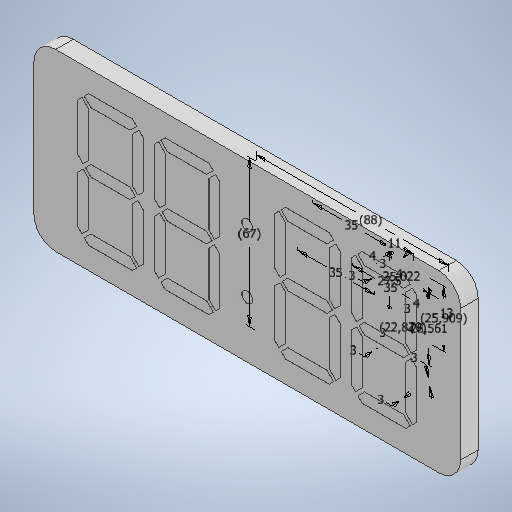
# Autodesk Inventor part: led 7 seg v3
Saved by Autodesk Inventor 2026 (Build 300175000, 175)
## iProperties
Created: 2025-05-20
Part Number: led 7 seg v3
Material: Generic
Document SubType Name: Modeling
Designer: Korobeynikov
Density: 1 g/cm^3
Appearance: Default
Author: Korobeynikov
Autodesk Inventor part; units mm, degrees
ref_plane "YZ Plane" through (0, 0, 0) normal (1, 0, 0) x (0, 1, 0)
ref_plane "XZ Plane" through (0, 0, 0) normal (0, 1, 0) x (-1, 0, 0)
ref_plane "XY Plane" through (0, 0, 0) normal (0, 0, 1) x (1, 0, 0)
sketch "Sketch1" plane through (0, 0, 0) normal (0, 0, 1) x (1, 0, 0)
  line L0 (-94.4527, 39.0647) -> (-94.5898, 54.9894)
  line L1 (-94.5898, 54.9894) -> (-92.9178, 56.6614)
  line L2 (-92.9178, 56.6614) -> (-89.7384, 53.6189)
  line L3 (-89.7384, 53.6189) -> (-89.5199, 39.1071)
  line L4 (-89.5199, 39.1071) -> (-91.8763, 36.6527)
  line L5 (-91.8763, 36.6527) -> (-94.4527, 39.0647)
  line L6 (-91.7267, 57.8164) -> (-89.9627, 59.534)
  line L7 (-89.9627, 59.534) -> (-75.9897, 59.6269)
  line L8 (-75.9897, 59.6269) -> (-74.3185, 57.8164)
  line L9 (-74.3185, 57.8164) -> (-77.2431, 54.8454)
  line L10 (-77.2431, 54.8454) -> (-88.6597, 54.6665)
  line L11 (-88.6597, 54.6665) -> (-91.7267, 57.8164)
  line L12 (-76.2169, 53.8075) -> (-73.4316, 57.0375)
  line L13 (-73.4316, 57.0375) -> (-71.7604, 55.4127)
  line L14 (-71.7604, 55.4127) -> (-71.1618, 39.5726)
  line L15 (-71.1618, 39.5726) -> (-73.39, 36.9729)
  line L16 (-73.39, 36.9729) -> (-75.9897, 39.3869)
  line L17 (-75.9897, 39.3869) -> (-76.2169, 53.8075)
  line L18 (-94.4164, 31.9932) -> (-91.951, 34.3514)
  line L19 (-91.951, 34.3514) -> (-89.4141, 31.9932)
  line L20 (-89.4141, 31.9932) -> (-89.2355, 17.2723)
  line L21 (-89.2355, 17.2723) -> (-92.344, 14.0208)
  line L22 (-92.344, 14.0208) -> (-94.4164, 15.5572)
  line L23 (-94.4164, 15.5572) -> (-94.4164, 31.9932)
  line L24 (-75.7293, 32.3505) -> (-73.4426, 34.7802)
  line L25 (-73.4426, 34.7802) -> (-71.1201, 32.3505)
  line L26 (-71.1201, 32.3505) -> (-70.5842, 16.4505)
  line L27 (-70.5842, 16.4505) -> (-72.2278, 14.4496)
  line L28 (-72.2278, 14.4496) -> (-75.4792, 17.5581)
  line L29 (-75.4792, 17.5581) -> (-75.7293, 32.3505)
  line L30 (-91.32, 13.0418) -> (-88.1993, 16.0932)
  line L31 (-88.1993, 16.0932) -> (-76.5869, 16.4862)
  line L32 (-76.5869, 16.4862) -> (-73.4783, 13.3777)
  line L33 (-73.4783, 13.3777) -> (-75.0147, 11.6269)
  line L34 (-75.0147, 11.6269) -> (-89.3605, 11.0378)
  line L35 (-89.3605, 11.0378) -> (-91.32, 13.0418)
  line L36 (-120.187, 34.9851) -> (-117.7903, 37.3494)
  line L37 (-117.7903, 37.3494) -> (-105.9036, 37.6409)
  line L38 (-105.9036, 37.6409) -> (-103.4421, 35.309)
  line L39 (-103.4421, 35.309) -> (-106.0008, 32.8474)
  line L40 (-106.0008, 32.8474) -> (-117.8069, 32.5723)
  line L41 (-117.8069, 32.5723) -> (-120.187, 34.9851)
  line L42 (-90.8505, 35.6062) -> (-88.4537, 37.9706)
  line L43 (-88.4537, 37.9706) -> (-76.5671, 38.2621)
  line L44 (-76.5671, 38.2621) -> (-74.1056, 35.9301)
  line L45 (-74.1056, 35.9301) -> (-76.6643, 33.4686)
  line L46 (-76.6643, 33.4686) -> (-88.4704, 33.1935)
  line L47 (-88.4704, 33.1935) -> (-90.8505, 35.6062)
  line L48 (-15, -30) -> (15, -30)
  line L49 (15, -30) -> (15, 30)
  line L50 (15, 30) -> (-15, 30)
  line L51 (-15, 30) -> (-15, -30)
  line L52 (-10, 30) -> (-10, -30)
  line L53 (10, 30) -> (10, -30)
  line L54 (-15, 25) -> (15, 25)
  line L55 (-15, -25) -> (15, -25)
  line L56 (-15, 2.5) -> (15, 2.5)
  line L57 (-15, -2.5) -> (15, -2.5)
  circle A0 centre (-12.5, 0) radius 1.0607
  line L58 (-11.4393, 0) -> (-8.9393, 2.5)
  line L59 (-11.4393, 0) -> (-8.9393, -2.5)
  line L60 (-12.5, 1.0607) -> (-15, 3.5607)
  line L61 (-12.5, 1.0607) -> (-10, 3.5607)
  line L62 (-12.5, -1.0607) -> (-15, -3.5607)
  line L63 (-12.5, -1.0607) -> (-10, -3.5607)
  line L64 (0, 8.5203) -> (0, -8.5203)
  line L65 (11.4393, 0) -> (8.9393, 2.5)
  line L66 (11.4393, 0) -> (8.9393, -2.5)
  line L67 (12.5, 1.0607) -> (15, 3.5607)
  line L68 (12.5, 1.0607) -> (10, 3.5607)
  line L69 (12.5, -1.0607) -> (15, -3.5607)
  line L70 (12.5, -1.0607) -> (10, -3.5607)
  line L71 (-15, 25) -> (-10, 30)
  line L72 (-15, 30) -> (-10, 25)
  line L73 (-13.0303, 26.9697) -> (-10, 23.9393)
  line L74 (-11.9697, 28.0303) -> (-8.9393, 25)
  line L75 (-6.2308, 0) -> (6.2308, 0)
  line L76 (13.0303, 26.9697) -> (10, 23.9393)
  line L77 (11.9697, 28.0303) -> (8.9393, 25)
  line L78 (-13.0303, -26.9697) -> (-10, -23.9393)
  line L79 (-11.9697, -28.0303) -> (-8.9393, -25)
  line L80 (13.0303, -26.9697) -> (10, -23.9393)
  line L81 (11.9697, -28.0303) -> (8.9393, -25)
  line L82 (10, 30) -> (15, 25)
  line L83 (-15, -25) -> (-10, -30)
  line L84 (10, -30) -> (15, -25)
  point P0 (0, 0)
  point P1 (-15, 0)
  point P2 (15, 0)
  point P3 (0, 0)
  dimension "d19" = 4.7815
  dimension "d20" = 48.4963
  dimension "d21" = 1.5036
  dimension "d22" = 20.0087
  dimension "d23" = 17.4083
  dimension "d24" = 22.8294
  dimension "d25" = 26.1583
  dimension "d26" = 4.8279
  dimension "d27" = 30
  dimension "d28" = 60
  dimension "d29" = 5
  dimension "d30" = 5
  dimension "d31" = 5
  dimension "d32" = 5
  dimension "d33" = 2.5
  dimension "d34" = 2.5
  dimension "d37" = 2.5
  dimension "d39" = 45
  dimension "d40" = 45
  dimension "d41" = 45
  dimension "d42" = 45
  dimension "d43" = 1.5
  dimension "d44" = 45
  dimension "d47" = 1.6712
  dimension "d50" = 0.75
  dimension "d51" = 0.75
  constraints: 168 end point, 21 symmetric about line, 17 point on line, 11 perpendicular, 3 horizontal alignment, 3 midpoint, 3 parallel, 3 point on circle, 2 horizontal, 2 vertical, 2 vertical alignment, 1 centre point, 1 coincident, 10 other
  measures "d19" vertical distance of L7.end L9.end
  measures "d20" vertical distance of L34.end L6.end
  measures "d21" distance of L10.end L2.end
  measures "d22" vertical distance of L4.end L1.end
  measures "d23" distance of L8.end L6.start
  measures "d24" horizontal distance of L13.end L0.end
  measures "d25" vertical distance of L7.end L45.end
  measures "d26" horizontal distance of L14.end L16.end
  measures "d27" distance of L50.end L49.end
  measures "d28" distance of L49.end L48.end
  measures "d30" distance between parallel lines of L49 L53
  measures "d31" distance between parallel lines of L50 L54
  measures "d32" distance between parallel lines of L48 L55
  measures "d33" distance from line of point (0, 0) L57
  measures "d34" distance from line of point (0, 0) L56
  measures "d37" distance of point (-15, 0) A0.centre
  measures "d39" angle of L57 L59
  measures "d40" angle of L56 L58
  measures "d41" angle to the sketch x axis of L60
  measures "d42" angle of L52 L61
  measures "d43" distance of L58.end L61.end
  measures "d44" angle to the sketch x axis of L62
  measures "d47" horizontal distance of L13.end L12.end
  measures "d50" distance between parallel lines of L72 L73
  measures "d51" distance between parallel lines of L74 L72
extrude "Extrusion1" add sketch "Sketch1" along normal blind 0.5 contours L52 L79 L55 L81 L53 L48 | L83 L79 L52 | L51 L62 L57 L63 L52 L78 L55 | L55 L78 L83 | L53 L81 L84 | L62 L63 L57 | L55 L80 L53 L70 L57 L69 L49 | L84 L80 L55 | L51 L54 L73 L52 L61 L56 L60 | L56 L61 L60 | L58 L52 L59 | L57 L70 L69 | L71 L73 L54 | L52 L58 L56 L64 L57 L59 | L64 L56 L65 L53 L66 L57 | L67 L56 L68 L53 L76 L54 L49 | L67 L68 L56 | L53 L65 L66 | L50 L53 L77 L54 L74 L52 | L52 L74 L71 | L54 L76 L82 | L82 L77 L53
pattern_linear "Rectangular Pattern1" count 2 spacing -35 along (-1, 0, 0) of "Extrusion1"
pattern_linear "Rectangular Pattern2" count 2 spacing 90 along (1, 0, 0) of "Extrusion1", "Rectangular Pattern1"
sketch "Sketch2" plane through (50, 3.5607, 0) normal (0, 0, -1) x (-1, 0, 0)
  line L0 (-25, 21.4393) -> (-25, 0) projected
  line L1 (-25, 10.7197) -> (0, 10.7197)
  line L2 (0, 0) -> (0, 21.4393) projected
  line L3 (-25, -7.1213) -> (-25, -28.5607) projected
  line L4 (-25, -17.841) -> (0, -17.841)
  line L5 (0, -28.5607) -> (0, -7.1213) projected
  circle A0 centre (-12.5, 10.7197) radius 2.5
  circle A1 centre (-12.5, -17.841) radius 2.5
  point P0 (50, -3.5607)
  dimension "d58" = 5
  dimension "d59" = 5
  dimension "d62" = 12.5
  constraints: 6 midpoint, 4 end point, 2 centre point
  measures "d58" diameter of A0
  measures "d59" diameter of A1
  measures "d62" distance from line of L2 A0.centre
extrude "Extrusion2" add sketch "Sketch2" against normal up to surface (0.5 mm away)
sketch "Sketch3" plane through (115, 30, 0.5) normal (0, 0, 1) x (1, 0, 0)
  line L0 (-140, 10) -> (35, 10)
  line L1 (45, 0) -> (45, -60)
  line L2 (35, -70) -> (-140, -70)
  line L3 (-150, -60) -> (-150, 0)
  line L4 (25, -26.4393) -> (25, -5) projected
  line L5 (-130, -5) -> (-130, -26.4393) projected
  line L6 (-105, 0) -> (-125, 0) projected
  line L7 (-125, -60) -> (-105, -60) projected
  arc A0 (-140, 10) -> (-150, 0) centre (-140, 0) ccw
  arc A1 (-150, -60) -> (-140, -70) centre (-140, -60) ccw
  arc A2 (45, 0) -> (35, 10) centre (35, 0) ccw
  arc A3 (35, -70) -> (45, -60) centre (35, -60) ccw
  line L8 (-103.0303, -1.9697) -> (-105, 0) projected
  line L9 (-105, 0) -> (-125, 0) projected
  line L10 (-125, 0) -> (-126.9697, -1.9697) projected
  line L11 (-126.9697, -1.9697) -> (-123.9393, -5) projected
  line L12 (-123.9393, -5) -> (-106.0607, -5) projected
  line L13 (-106.0607, -5) -> (-103.0303, -1.9697) projected
  line L14 (-128.0303, -3.0303) -> (-130, -5) projected
  line L15 (-130, -5) -> (-130, -26.4393) projected
  line L16 (-130, -26.4393) -> (-127.5, -28.9393) projected
  line L17 (-127.5, -28.9393) -> (-125, -26.4393) projected
  line L18 (-125, -26.4393) -> (-125, -6.0607) projected
  line L19 (-125, -6.0607) -> (-128.0303, -3.0303) projected
  line L20 (-123.9393, -27.5) -> (-126.4393, -30) projected
  line L21 (-126.4393, -30) -> (-123.9393, -32.5) projected
  line L22 (-123.9393, -32.5) -> (-106.0607, -32.5) projected
  line L23 (-106.0607, -32.5) -> (-103.5607, -30) projected
  line L24 (-103.5607, -30) -> (-106.0607, -27.5) projected
  line L25 (-106.0607, -27.5) -> (-123.9393, -27.5) projected
  line L26 (-125, -53.9393) -> (-125, -33.5607) projected
  line L27 (-130, -33.5607) -> (-130, -55) projected
  line L28 (-125, -53.9393) -> (-125, -33.5607) projected
  line L29 (-125, -33.5607) -> (-127.5, -31.0607) projected
  line L30 (-127.5, -31.0607) -> (-130, -33.5607) projected
  line L31 (-130, -33.5607) -> (-130, -55) projected
  line L32 (-130, -55) -> (-128.0303, -56.9697) projected
  line L33 (-128.0303, -56.9697) -> (-125, -53.9393) projected
  line L34 (-106.0607, -55) -> (-123.9393, -55) projected
  line L35 (-106.0607, -55) -> (-123.9393, -55) projected
  line L36 (-123.9393, -55) -> (-126.9697, -58.0303) projected
  line L37 (-126.9697, -58.0303) -> (-125, -60) projected
  line L38 (-125, -60) -> (-105, -60) projected
  line L39 (-105, -60) -> (-103.0303, -58.0303) projected
  line L40 (-103.0303, -58.0303) -> (-106.0607, -55) projected
  line L41 (-101.9697, -56.9697) -> (-100, -55) projected
  line L42 (-100, -55) -> (-100, -33.5607) projected
  line L43 (-100, -33.5607) -> (-102.5, -31.0607) projected
  line L44 (-102.5, -31.0607) -> (-105, -33.5607) projected
  line L45 (-105, -33.5607) -> (-105, -53.9393) projected
  line L46 (-105, -53.9393) -> (-101.9697, -56.9697) projected
  line L47 (-105, -6.0607) -> (-105, -26.4393) projected
  line L48 (-105, -26.4393) -> (-102.5, -28.9393) projected
  line L49 (-102.5, -28.9393) -> (-100, -26.4393) projected
  line L50 (-100, -26.4393) -> (-100, -5) projected
  line L51 (-100, -5) -> (-101.9697, -3.0303) projected
  line L52 (-101.9697, -3.0303) -> (-105, -6.0607) projected
  line L53 (-90, -26.4393) -> (-90, -6.0607) projected
  line L54 (-93.0303, -3.0303) -> (-95, -5) projected
  line L55 (-95, -5) -> (-95, -26.4393) projected
  line L56 (-95, -26.4393) -> (-92.5, -28.9393) projected
  line L57 (-92.5, -28.9393) -> (-90, -26.4393) projected
  line L58 (-90, -26.4393) -> (-90, -6.0607) projected
  line L59 (-90, -6.0607) -> (-93.0303, -3.0303) projected
  line L60 (-68.0303, -1.9697) -> (-70, 0) projected
  line L61 (-70, 0) -> (-90, 0) projected
  line L62 (-90, 0) -> (-91.9697, -1.9697) projected
  line L63 (-91.9697, -1.9697) -> (-88.9393, -5) projected
  line L64 (-88.9393, -5) -> (-71.0607, -5) projected
  line L65 (-71.0607, -5) -> (-68.0303, -1.9697) projected
  line L66 (-70, -6.0607) -> (-70, -26.4393) projected
  line L67 (-70, -26.4393) -> (-67.5, -28.9393) projected
  line L68 (-67.5, -28.9393) -> (-65, -26.4393) projected
  line L69 (-65, -26.4393) -> (-65, -5) projected
  line L70 (-65, -5) -> (-66.9697, -3.0303) projected
  line L71 (-66.9697, -3.0303) -> (-70, -6.0607) projected
  line L72 (-88.9393, -27.5) -> (-91.4393, -30) projected
  line L73 (-91.4393, -30) -> (-88.9393, -32.5) projected
  line L74 (-88.9393, -32.5) -> (-71.0607, -32.5) projected
  line L75 (-71.0607, -32.5) -> (-68.5607, -30) projected
  line L76 (-68.5607, -30) -> (-71.0607, -27.5) projected
  line L77 (-71.0607, -27.5) -> (-88.9393, -27.5) projected
  line L78 (-95, -33.5607) -> (-95, -55) projected
  line L79 (-90, -53.9393) -> (-90, -33.5607) projected
  line L80 (-90, -33.5607) -> (-92.5, -31.0607) projected
  line L81 (-92.5, -31.0607) -> (-95, -33.5607) projected
  line L82 (-95, -33.5607) -> (-95, -55) projected
  line L83 (-95, -55) -> (-93.0303, -56.9697) projected
  line L84 (-93.0303, -56.9697) -> (-90, -53.9393) projected
  line L85 (-66.9697, -56.9697) -> (-65, -55) projected
  line L86 (-65, -55) -> (-65, -33.5607) projected
  line L87 (-65, -33.5607) -> (-67.5, -31.0607) projected
  line L88 (-67.5, -31.0607) -> (-70, -33.5607) projected
  line L89 (-70, -33.5607) -> (-70, -53.9393) projected
  line L90 (-70, -53.9393) -> (-66.9697, -56.9697) projected
  line L91 (-71.0607, -55) -> (-88.9393, -55) projected
  line L92 (-88.9393, -55) -> (-91.9697, -58.0303) projected
  line L93 (-91.9697, -58.0303) -> (-90, -60) projected
  line L94 (-90, -60) -> (-70, -60) projected
  line L95 (-70, -60) -> (-68.0303, -58.0303) projected
  line L96 (-68.0303, -58.0303) -> (-71.0607, -55) projected
  circle A4 centre (-52.5, -44.2803) radius 2.5 projected
  circle A5 centre (-52.5, -15.7197) radius 2.5 projected
  line L97 (-40, -5) -> (-40, -26.4393) projected
  line L98 (-13.0303, -1.9697) -> (-15, 0) projected
  line L99 (-15, 0) -> (-35, 0) projected
  line L100 (-35, 0) -> (-36.9697, -1.9697) projected
  line L101 (-36.9697, -1.9697) -> (-33.9393, -5) projected
  line L102 (-33.9393, -5) -> (-16.0607, -5) projected
  line L103 (-16.0607, -5) -> (-13.0303, -1.9697) projected
  line L104 (-15, -6.0607) -> (-15, -26.4393) projected
  line L105 (-15, -26.4393) -> (-12.5, -28.9393) projected
  line L106 (-12.5, -28.9393) -> (-10, -26.4393) projected
  line L107 (-10, -26.4393) -> (-10, -5) projected
  line L108 (-10, -5) -> (-11.9697, -3.0303) projected
  line L109 (-11.9697, -3.0303) -> (-15, -6.0607) projected
  line L110 (-38.0303, -3.0303) -> (-40, -5) projected
  line L111 (-40, -5) -> (-40, -26.4393) projected
  line L112 (-40, -26.4393) -> (-37.5, -28.9393) projected
  line L113 (-37.5, -28.9393) -> (-35, -26.4393) projected
  line L114 (-35, -26.4393) -> (-35, -6.0607) projected
  line L115 (-35, -6.0607) -> (-38.0303, -3.0303) projected
  line L116 (-33.9393, -27.5) -> (-36.4393, -30) projected
  line L117 (-36.4393, -30) -> (-33.9393, -32.5) projected
  line L118 (-33.9393, -32.5) -> (-16.0607, -32.5) projected
  line L119 (-16.0607, -32.5) -> (-13.5607, -30) projected
  line L120 (-13.5607, -30) -> (-16.0607, -27.5) projected
  line L121 (-16.0607, -27.5) -> (-33.9393, -27.5) projected
  line L122 (-35, -53.9393) -> (-35, -33.5607) projected
  line L123 (-35, -33.5607) -> (-37.5, -31.0607) projected
  line L124 (-37.5, -31.0607) -> (-40, -33.5607) projected
  line L125 (-40, -33.5607) -> (-40, -55) projected
  line L126 (-40, -55) -> (-38.0303, -56.9697) projected
  line L127 (-38.0303, -56.9697) -> (-35, -53.9393) projected
  line L128 (-16.0607, -55) -> (-33.9393, -55) projected
  line L129 (-33.9393, -55) -> (-36.9697, -58.0303) projected
  line L130 (-36.9697, -58.0303) -> (-35, -60) projected
  line L131 (-35, -60) -> (-15, -60) projected
  line L132 (-15, -60) -> (-13.0303, -58.0303) projected
  line L133 (-13.0303, -58.0303) -> (-16.0607, -55) projected
  line L134 (-11.9697, -56.9697) -> (-10, -55) projected
  line L135 (-10, -55) -> (-10, -33.5607) projected
  line L136 (-10, -33.5607) -> (-12.5, -31.0607) projected
  line L137 (-12.5, -31.0607) -> (-15, -33.5607) projected
  line L138 (-15, -33.5607) -> (-15, -53.9393) projected
  line L139 (-15, -53.9393) -> (-11.9697, -56.9697) projected
  line L140 (0, -53.9393) -> (0, -33.5607) projected
  line L141 (0, -33.5607) -> (-2.5, -31.0607) projected
  line L142 (-2.5, -31.0607) -> (-5, -33.5607) projected
  line L143 (-5, -33.5607) -> (-5, -55) projected
  line L144 (-5, -55) -> (-3.0303, -56.9697) projected
  line L145 (-3.0303, -56.9697) -> (0, -53.9393) projected
  line L146 (1.0607, -27.5) -> (-1.4393, -30) projected
  line L147 (-1.4393, -30) -> (1.0607, -32.5) projected
  line L148 (1.0607, -32.5) -> (18.9393, -32.5) projected
  line L149 (18.9393, -32.5) -> (21.4393, -30) projected
  line L150 (21.4393, -30) -> (18.9393, -27.5) projected
  line L151 (18.9393, -27.5) -> (1.0607, -27.5) projected
  line L152 (-3.0303, -3.0303) -> (-5, -5) projected
  line L153 (-5, -5) -> (-5, -26.4393) projected
  line L154 (-5, -26.4393) -> (-2.5, -28.9393) projected
  line L155 (-2.5, -28.9393) -> (0, -26.4393) projected
  line L156 (0, -26.4393) -> (0, -6.0607) projected
  line L157 (0, -6.0607) -> (-3.0303, -3.0303) projected
  line L158 (21.9697, -1.9697) -> (20, 0) projected
  line L159 (20, 0) -> (0, 0) projected
  line L160 (0, 0) -> (-1.9697, -1.9697) projected
  line L161 (-1.9697, -1.9697) -> (1.0607, -5) projected
  line L162 (1.0607, -5) -> (18.9393, -5) projected
  line L163 (18.9393, -5) -> (21.9697, -1.9697) projected
  line L164 (20, -6.0607) -> (20, -26.4393) projected
  line L165 (20, -26.4393) -> (22.5, -28.9393) projected
  line L166 (22.5, -28.9393) -> (25, -26.4393) projected
  line L167 (25, -26.4393) -> (25, -5) projected
  line L168 (25, -5) -> (23.0303, -3.0303) projected
  line L169 (23.0303, -3.0303) -> (20, -6.0607) projected
  line L170 (23.0303, -56.9697) -> (25, -55) projected
  line L171 (25, -55) -> (25, -33.5607) projected
  line L172 (25, -33.5607) -> (22.5, -31.0607) projected
  line L173 (22.5, -31.0607) -> (20, -33.5607) projected
  line L174 (20, -33.5607) -> (20, -53.9393) projected
  line L175 (20, -53.9393) -> (23.0303, -56.9697) projected
  line L176 (18.9393, -55) -> (1.0607, -55) projected
  line L177 (1.0607, -55) -> (-1.9697, -58.0303) projected
  line L178 (-1.9697, -58.0303) -> (0, -60) projected
  line L179 (0, -60) -> (20, -60) projected
  line L180 (20, -60) -> (21.9697, -58.0303) projected
  line L181 (21.9697, -58.0303) -> (18.9393, -55) projected
  point P0 (-115, -30)
  dimension "d63" = 20
  dimension "d64" = 20
  dimension "d65" = 10
  dimension "d66" = 10
  dimension "d67" = 10
  dimension "d68" = 10
  constraints: 8 end point, 8 point on circle, 8 tangent, 4 centre point, 2 equal radius, 2 parallel, 1 horizontal, 1 perpendicular
  measures "d63" distance between parallel lines of L1 L4
  measures "d64" distance between parallel lines of L3 L5
  measures "d65" distance between parallel lines of L6 L0
  measures "d66" distance between parallel lines of L2 L7
  measures "d67" radius of A0
  measures "d68" radius of A1
extrude "Extrusion3" add sketch "Sketch3" along normal blind 0.05 and the other way blind 8
sketch "Sketch4" plane through (115, 30, -7.5) normal (0, 0, -1) x (-1, 0, 0)
  line L0 (-35, -70) -> (140, -70) projected
  arc A0 (140, -70) -> (150, -60) centre (140, -60) ccw projected
  line L1 (150, -60) -> (150, 0) projected
  arc A1 (150, 0) -> (140, 10) centre (140, 0) ccw projected
  line L2 (140, 10) -> (-35, 10) projected
  arc A2 (-35, 10) -> (-45, 0) centre (-35, 0) ccw projected
  line L3 (-45, 0) -> (-45, -60) projected
  arc A3 (-45, -60) -> (-35, -70) centre (-35, -60) ccw projected
  circle A4 centre (52.5, -15.7197) radius 2.5 projected
  line L4 (-22.5, -28.9393) -> (-25, -26.4393) projected
  line L5 (-25, -26.4393) -> (-25, -5) projected
  line L6 (-25, -5) -> (-23.0303, -3.0303) projected
  line L7 (-23.0303, -3.0303) -> (-20, -6.0607) projected
  line L8 (-20, -6.0607) -> (-20, -26.4393) projected
  line L9 (-20, -26.4393) -> (-22.5, -28.9393) projected
  line L10 (128.0303, -3.0303) -> (130, -5) projected
  line L11 (130, -5) -> (130, -26.4393) projected
  line L12 (130, -26.4393) -> (127.5, -28.9393) projected
  line L13 (127.5, -28.9393) -> (125, -26.4393) projected
  line L14 (125, -26.4393) -> (125, -6.0607) projected
  line L15 (125, -6.0607) -> (128.0303, -3.0303) projected
  line L16 (103.0303, -1.9697) -> (105, 0) projected
  line L17 (105, 0) -> (125, 0) projected
  line L18 (125, 0) -> (126.9697, -1.9697) projected
  line L19 (126.9697, -1.9697) -> (123.9393, -5) projected
  line L20 (123.9393, -5) -> (106.0607, -5) projected
  line L21 (106.0607, -5) -> (103.0303, -1.9697) projected
  line L22 (126.9697, -58.0303) -> (125, -60) projected
  line L23 (125, -60) -> (105, -60) projected
  line L24 (105, -60) -> (103.0303, -58.0303) projected
  line L25 (103.0303, -58.0303) -> (106.0607, -55) projected
  line L26 (106.0607, -55) -> (123.9393, -55) projected
  line L27 (123.9393, -55) -> (126.9697, -58.0303) projected
  line L28 (127.5, -31.0607) -> (130, -33.5607) projected
  line L29 (130, -33.5607) -> (130, -55) projected
  line L30 (130, -55) -> (128.0303, -56.9697) projected
  line L31 (128.0303, -56.9697) -> (125, -53.9393) projected
  line L32 (125, -53.9393) -> (125, -33.5607) projected
  line L33 (125, -33.5607) -> (127.5, -31.0607) projected
  line L34 (92.5, -28.9393) -> (90, -26.4393) projected
  line L35 (90, -26.4393) -> (90, -6.0607) projected
  line L36 (90, -6.0607) -> (93.0303, -3.0303) projected
  line L37 (93.0303, -3.0303) -> (95, -5) projected
  line L38 (95, -5) -> (95, -26.4393) projected
  line L39 (95, -26.4393) -> (92.5, -28.9393) projected
  line L40 (92.5, -31.0607) -> (95, -33.5607) projected
  line L41 (95, -33.5607) -> (95, -55) projected
  line L42 (95, -55) -> (93.0303, -56.9697) projected
  line L43 (93.0303, -56.9697) -> (90, -53.9393) projected
  line L44 (90, -53.9393) -> (90, -33.5607) projected
  line L45 (90, -33.5607) -> (92.5, -31.0607) projected
  circle A5 centre (52.5, -44.2803) radius 2.5 projected
  line L46 (38.0303, -3.0303) -> (40, -5) projected
  line L47 (40, -5) -> (40, -26.4393) projected
  line L48 (40, -26.4393) -> (37.5, -28.9393) projected
  line L49 (37.5, -28.9393) -> (35, -26.4393) projected
  line L50 (35, -26.4393) -> (35, -6.0607) projected
  line L51 (35, -6.0607) -> (38.0303, -3.0303) projected
  line L52 (-21.9697, -58.0303) -> (-18.9393, -55) projected
  line L53 (-18.9393, -55) -> (-1.0607, -55) projected
  line L54 (-1.0607, -55) -> (1.9697, -58.0303) projected
  line L55 (1.9697, -58.0303) -> (0, -60) projected
  line L56 (0, -60) -> (-20, -60) projected
  line L57 (-20, -60) -> (-21.9697, -58.0303) projected
  line L58 (-20, -53.9393) -> (-23.0303, -56.9697) projected
  line L59 (-23.0303, -56.9697) -> (-25, -55) projected
  line L60 (-25, -55) -> (-25, -33.5607) projected
  line L61 (-25, -33.5607) -> (-22.5, -31.0607) projected
  line L62 (-22.5, -31.0607) -> (-20, -33.5607) projected
  line L63 (-20, -33.5607) -> (-20, -53.9393) projected
  line L64 (-18.9393, -5) -> (-21.9697, -1.9697) projected
  line L65 (-21.9697, -1.9697) -> (-20, 0) projected
  line L66 (-20, 0) -> (0, 0) projected
  line L67 (0, 0) -> (1.9697, -1.9697) projected
  line L68 (1.9697, -1.9697) -> (-1.0607, -5) projected
  line L69 (-1.0607, -5) -> (-18.9393, -5) projected
  line L70 (0, -6.0607) -> (3.0303, -3.0303) projected
  line L71 (3.0303, -3.0303) -> (5, -5) projected
  line L72 (5, -5) -> (5, -26.4393) projected
  line L73 (5, -26.4393) -> (2.5, -28.9393) projected
  line L74 (2.5, -28.9393) -> (0, -26.4393) projected
  line L75 (0, -26.4393) -> (0, -6.0607) projected
  line L76 (-18.9393, -27.5) -> (-1.0607, -27.5) projected
  line L77 (-1.0607, -27.5) -> (1.4393, -30) projected
  line L78 (1.4393, -30) -> (-1.0607, -32.5) projected
  line L79 (-1.0607, -32.5) -> (-18.9393, -32.5) projected
  line L80 (-18.9393, -32.5) -> (-21.4393, -30) projected
  line L81 (-21.4393, -30) -> (-18.9393, -27.5) projected
  line L82 (3.0303, -56.9697) -> (0, -53.9393) projected
  line L83 (0, -53.9393) -> (0, -33.5607) projected
  line L84 (0, -33.5607) -> (2.5, -31.0607) projected
  line L85 (2.5, -31.0607) -> (5, -33.5607) projected
  line L86 (5, -33.5607) -> (5, -55) projected
  line L87 (5, -55) -> (3.0303, -56.9697) projected
  line L88 (15, -53.9393) -> (11.9697, -56.9697) projected
  line L89 (11.9697, -56.9697) -> (10, -55) projected
  line L90 (10, -55) -> (10, -33.5607) projected
  line L91 (10, -33.5607) -> (12.5, -31.0607) projected
  line L92 (12.5, -31.0607) -> (15, -33.5607) projected
  line L93 (15, -33.5607) -> (15, -53.9393) projected
  line L94 (13.0303, -58.0303) -> (16.0607, -55) projected
  line L95 (16.0607, -55) -> (33.9393, -55) projected
  line L96 (33.9393, -55) -> (36.9697, -58.0303) projected
  line L97 (36.9697, -58.0303) -> (35, -60) projected
  line L98 (35, -60) -> (15, -60) projected
  line L99 (15, -60) -> (13.0303, -58.0303) projected
  line L100 (38.0303, -56.9697) -> (35, -53.9393) projected
  line L101 (35, -53.9393) -> (35, -33.5607) projected
  line L102 (35, -33.5607) -> (37.5, -31.0607) projected
  line L103 (37.5, -31.0607) -> (40, -33.5607) projected
  line L104 (40, -33.5607) -> (40, -55) projected
  line L105 (40, -55) -> (38.0303, -56.9697) projected
  line L106 (16.0607, -27.5) -> (33.9393, -27.5) projected
  line L107 (33.9393, -27.5) -> (36.4393, -30) projected
  line L108 (36.4393, -30) -> (33.9393, -32.5) projected
  line L109 (33.9393, -32.5) -> (16.0607, -32.5) projected
  line L110 (16.0607, -32.5) -> (13.5607, -30) projected
  line L111 (13.5607, -30) -> (16.0607, -27.5) projected
  line L112 (11.9697, -3.0303) -> (15, -6.0607) projected
  line L113 (15, -6.0607) -> (15, -26.4393) projected
  line L114 (15, -26.4393) -> (12.5, -28.9393) projected
  line L115 (12.5, -28.9393) -> (10, -26.4393) projected
  line L116 (10, -26.4393) -> (10, -5) projected
  line L117 (10, -5) -> (11.9697, -3.0303) projected
  line L118 (16.0607, -5) -> (13.0303, -1.9697) projected
  line L119 (13.0303, -1.9697) -> (15, 0) projected
  line L120 (15, 0) -> (35, 0) projected
  line L121 (35, 0) -> (36.9697, -1.9697) projected
  line L122 (36.9697, -1.9697) -> (33.9393, -5) projected
  line L123 (33.9393, -5) -> (16.0607, -5) projected
  line L124 (68.0303, -58.0303) -> (71.0607, -55) projected
  line L125 (71.0607, -55) -> (88.9393, -55) projected
  line L126 (88.9393, -55) -> (91.9697, -58.0303) projected
  line L127 (91.9697, -58.0303) -> (90, -60) projected
  line L128 (90, -60) -> (70, -60) projected
  line L129 (70, -60) -> (68.0303, -58.0303) projected
  line L130 (70, -53.9393) -> (66.9697, -56.9697) projected
  line L131 (66.9697, -56.9697) -> (65, -55) projected
  line L132 (65, -55) -> (65, -33.5607) projected
  line L133 (65, -33.5607) -> (67.5, -31.0607) projected
  line L134 (67.5, -31.0607) -> (70, -33.5607) projected
  line L135 (70, -33.5607) -> (70, -53.9393) projected
  line L136 (71.0607, -27.5) -> (88.9393, -27.5) projected
  line L137 (88.9393, -27.5) -> (91.4393, -30) projected
  line L138 (91.4393, -30) -> (88.9393, -32.5) projected
  line L139 (88.9393, -32.5) -> (71.0607, -32.5) projected
  line L140 (71.0607, -32.5) -> (68.5607, -30) projected
  line L141 (68.5607, -30) -> (71.0607, -27.5) projected
  line L142 (66.9697, -3.0303) -> (70, -6.0607) projected
  line L143 (70, -6.0607) -> (70, -26.4393) projected
  line L144 (70, -26.4393) -> (67.5, -28.9393) projected
  line L145 (67.5, -28.9393) -> (65, -26.4393) projected
  line L146 (65, -26.4393) -> (65, -5) projected
  line L147 (65, -5) -> (66.9697, -3.0303) projected
  line L148 (71.0607, -5) -> (68.0303, -1.9697) projected
  line L149 (68.0303, -1.9697) -> (70, 0) projected
  line L150 (70, 0) -> (90, 0) projected
  line L151 (90, 0) -> (91.9697, -1.9697) projected
  line L152 (91.9697, -1.9697) -> (88.9393, -5) projected
  line L153 (88.9393, -5) -> (71.0607, -5) projected
  line L154 (101.9697, -3.0303) -> (105, -6.0607) projected
  line L155 (105, -6.0607) -> (105, -26.4393) projected
  line L156 (105, -26.4393) -> (102.5, -28.9393) projected
  line L157 (102.5, -28.9393) -> (100, -26.4393) projected
  line L158 (100, -26.4393) -> (100, -5) projected
  line L159 (100, -5) -> (101.9697, -3.0303) projected
  line L160 (105, -53.9393) -> (101.9697, -56.9697) projected
  line L161 (101.9697, -56.9697) -> (100, -55) projected
  line L162 (100, -55) -> (100, -33.5607) projected
  line L163 (100, -33.5607) -> (102.5, -31.0607) projected
  line L164 (102.5, -31.0607) -> (105, -33.5607) projected
  line L165 (105, -33.5607) -> (105, -53.9393) projected
  line L166 (106.0607, -27.5) -> (123.9393, -27.5) projected
  line L167 (123.9393, -27.5) -> (126.4393, -30) projected
  line L168 (126.4393, -30) -> (123.9393, -32.5) projected
  line L169 (123.9393, -32.5) -> (106.0607, -32.5) projected
  line L170 (106.0607, -32.5) -> (103.5607, -30) projected
  line L171 (103.5607, -30) -> (106.0607, -27.5) projected
  line L172 (-35, 8) -> (140, 8)
  arc A6 (148, 0) -> (140, 8) centre (140, 0) ccw
  line L173 (148, 0) -> (148, -60)
  arc A7 (140, -68) -> (148, -60) centre (140, -60) ccw
  line L174 (140, -68) -> (-35, -68)
  arc A8 (-43, -60) -> (-35, -68) centre (-35, -60) ccw
  line L175 (-43, -60) -> (-43, 0)
  arc A9 (-35, 8) -> (-43, 0) centre (-35, 0) ccw
  line L176 (-20, -5) -> (0, -5)
  line L177 (0, -5) -> (0, -27.5)
  line L178 (0, -27.5) -> (-20, -27.5)
  line L179 (-20, -27.5) -> (-20, -5)
  line L180 (-20, -32.5) -> (0, -32.5)
  line L181 (0, -32.5) -> (0, -55)
  line L182 (0, -55) -> (-20, -55)
  line L183 (-20, -55) -> (-20, -32.5)
  line L184 (-18.5, -6.5) -> (-1.5, -6.5)
  line L185 (-1.5, -6.5) -> (-1.5, -26)
  line L186 (-1.5, -26) -> (-18.5, -26)
  line L187 (-18.5, -26) -> (-18.5, -6.5)
  line L188 (-1.5, -34) -> (-18.5, -34)
  line L189 (-18.5, -34) -> (-18.5, -53.5)
  line L190 (-18.5, -53.5) -> (-1.5, -53.5)
  line L191 (-1.5, -53.5) -> (-1.5, -34)
  line L192 (16.5, -6.5) -> (33.5, -6.5)
  line L193 (16.5, -26) -> (16.5, -6.5)
  line L194 (33.5, -6.5) -> (33.5, -26)
  line L195 (33.5, -26) -> (16.5, -26)
  line L196 (33.5, -34) -> (16.5, -34)
  line L197 (16.5, -34) -> (16.5, -53.5)
  line L198 (33.5, -53.5) -> (33.5, -34)
  line L199 (16.5, -53.5) -> (33.5, -53.5)
  line L200 (71.5, -26) -> (71.5, -6.5)
  line L201 (71.5, -6.5) -> (88.5, -6.5)
  line L202 (88.5, -6.5) -> (88.5, -26)
  line L203 (88.5, -26) -> (71.5, -26)
  line L204 (88.5, -34) -> (71.5, -34)
  line L205 (71.5, -34) -> (71.5, -53.5)
  line L206 (88.5, -53.5) -> (88.5, -34)
  line L207 (71.5, -53.5) -> (88.5, -53.5)
  line L208 (106.5, -26) -> (106.5, -6.5)
  line L209 (106.5, -6.5) -> (123.5, -6.5)
  line L210 (123.5, -6.5) -> (123.5, -26)
  line L211 (123.5, -26) -> (106.5, -26)
  line L212 (123.5, -34) -> (106.5, -34)
  line L213 (123.5, -53.5) -> (123.5, -34)
  line L214 (106.5, -34) -> (106.5, -53.5)
  line L215 (106.5, -53.5) -> (123.5, -53.5)
  line L216 (-25, 0) -> (40, 0)
  line L217 (40, 0) -> (40, -60)
  line L218 (40, -60) -> (-25, -60)
  line L219 (-25, -60) -> (-25, 0)
  line L220 (41.5, 1.5) -> (-26.5, 1.5)
  line L221 (-26.5, 1.5) -> (-26.5, -61.5)
  line L222 (-26.5, -61.5) -> (41.5, -61.5)
  line L223 (41.5, -61.5) -> (41.5, 1.5)
  line L224 (131.5, 1.5) -> (63.5, 1.5)
  line L225 (63.5, 1.5) -> (63.5, -61.5)
  line L226 (131.5, -61.5) -> (131.5, 1.5)
  line L227 (63.5, -61.5) -> (131.5, -61.5)
  circle A10 centre (52.5, -15.7197) radius 4
  circle A11 centre (52.5, -44.2803) radius 4
  point P0 (115, -30)
  dimension "d73" = 2
  dimension "d75" = 1.5
  dimension "d76" = 1.5
  dimension "d79" = 35
  dimension "d86" = 90
  dimension "d92" = 1.5
  dimension "d95" = 90
  dimension "d100" = 1.5
  dimension "d101" = 1.5
  constraints: 112 end point, 12 parallel, 8 point on circle, 6 centre point, 6 horizontal, 6 perpendicular, 3 point on line, 2 collinear, 70 other
  measures "d73" distance between parallel lines of L2 L172
  measures "d75" distance between parallel lines of L179 L187
  measures "d76" distance between parallel lines of L180 L188
  measures "d79" distance of L184.start L192.start
  measures "d86" distance of L186.end L200.start
  measures "d92" distance between parallel lines of L216 L220
  measures "d95" distance of L220.start L224.start
  measures "d100" radial gap between concentric circles of A4 A10
  measures "d101" radial gap between concentric circles of A5 A11
extrude "Extrusion4" cut sketch "Sketch4" against normal blind 7 contours L172 A6 L173 A7 L174 A8 L175 A9 | L184 L185 L186 L187 | L191 L190 L189 L188 | L192 L194 L195 L193 | L198 L199 L197 L196 | L200 L201 L202 L203 | L206 L207 L205 L204 | L208 L209 L210 L211 | L213 L215 L214 L212
sketch "Sketch5" plane through (115, 30, -7.5) normal (0, 0, -1) x (-1, 0, 0)
  line L0 (-1.5, -53.5) -> (-18.5, -53.5) projected
  line L1 (-18.5, -53.5) -> (-18.5, -34) projected
  line L2 (-18.5, -34) -> (-1.5, -34) projected
  line L3 (-1.5, -34) -> (-1.5, -53.5) projected
  line L4 (33.5, -53.5) -> (16.5, -53.5) projected
  line L5 (16.5, -53.5) -> (16.5, -34) projected
  line L6 (16.5, -34) -> (33.5, -34) projected
  line L7 (33.5, -34) -> (33.5, -53.5) projected
  line L8 (-1.5, -6.5) -> (-1.5, -26) projected
  line L9 (-1.5, -26) -> (-18.5, -26) projected
  line L10 (-18.5, -26) -> (-18.5, -6.5) projected
  line L11 (-18.5, -6.5) -> (-1.5, -6.5) projected
  line L12 (33.5, -6.5) -> (33.5, -26) projected
  line L13 (33.5, -26) -> (16.5, -26) projected
  line L14 (16.5, -26) -> (16.5, -6.5) projected
  line L15 (16.5, -6.5) -> (33.5, -6.5) projected
  line L16 (-26.5, -61.5) -> (41.5, -61.5) projected
  line L17 (41.5, -61.5) -> (41.5, 1.5) projected
  line L18 (41.5, 1.5) -> (-26.5, 1.5) projected
  line L19 (-26.5, 1.5) -> (-26.5, -61.5) projected
  line L20 (-22.5, -28.9393) -> (-25, -26.4393) projected
  line L21 (-25, -26.4393) -> (-25, -5) projected
  line L22 (-25, -5) -> (-23.0303, -3.0303) projected
  line L23 (-23.0303, -3.0303) -> (-20, -6.0607) projected
  line L24 (-20, -6.0607) -> (-20, -26.4393) projected
  line L25 (-20, -26.4393) -> (-22.5, -28.9393) projected
  line L26 (38.0303, -3.0303) -> (40, -5) projected
  line L27 (40, -5) -> (40, -26.4393) projected
  line L28 (40, -26.4393) -> (37.5, -28.9393) projected
  line L29 (37.5, -28.9393) -> (35, -26.4393) projected
  line L30 (35, -26.4393) -> (35, -6.0607) projected
  line L31 (35, -6.0607) -> (38.0303, -3.0303) projected
  line L32 (-21.9697, -58.0303) -> (-18.9393, -55) projected
  line L33 (-18.9393, -55) -> (-1.0607, -55) projected
  line L34 (-1.0607, -55) -> (1.9697, -58.0303) projected
  line L35 (1.9697, -58.0303) -> (0, -60) projected
  line L36 (0, -60) -> (-20, -60) projected
  line L37 (-20, -60) -> (-21.9697, -58.0303) projected
  line L38 (-20, -53.9393) -> (-23.0303, -56.9697) projected
  line L39 (-23.0303, -56.9697) -> (-25, -55) projected
  line L40 (-25, -55) -> (-25, -33.5607) projected
  line L41 (-25, -33.5607) -> (-22.5, -31.0607) projected
  line L42 (-22.5, -31.0607) -> (-20, -33.5607) projected
  line L43 (-20, -33.5607) -> (-20, -53.9393) projected
  line L44 (-18.9393, -5) -> (-21.9697, -1.9697) projected
  line L45 (-21.9697, -1.9697) -> (-20, 0) projected
  line L46 (-20, 0) -> (0, 0) projected
  line L47 (0, 0) -> (1.9697, -1.9697) projected
  line L48 (1.9697, -1.9697) -> (-1.0607, -5) projected
  line L49 (-1.0607, -5) -> (-18.9393, -5) projected
  line L50 (0, -6.0607) -> (3.0303, -3.0303) projected
  line L51 (3.0303, -3.0303) -> (5, -5) projected
  line L52 (5, -5) -> (5, -26.4393) projected
  line L53 (5, -26.4393) -> (2.5, -28.9393) projected
  line L54 (2.5, -28.9393) -> (0, -26.4393) projected
  line L55 (0, -26.4393) -> (0, -6.0607) projected
  line L56 (-18.9393, -27.5) -> (-1.0607, -27.5) projected
  line L57 (-1.0607, -27.5) -> (1.4393, -30) projected
  line L58 (1.4393, -30) -> (-1.0607, -32.5) projected
  line L59 (-1.0607, -32.5) -> (-18.9393, -32.5) projected
  line L60 (-18.9393, -32.5) -> (-21.4393, -30) projected
  line L61 (-21.4393, -30) -> (-18.9393, -27.5) projected
  line L62 (3.0303, -56.9697) -> (0, -53.9393) projected
  line L63 (0, -53.9393) -> (0, -33.5607) projected
  line L64 (0, -33.5607) -> (2.5, -31.0607) projected
  line L65 (2.5, -31.0607) -> (5, -33.5607) projected
  line L66 (5, -33.5607) -> (5, -55) projected
  line L67 (5, -55) -> (3.0303, -56.9697) projected
  line L68 (15, -53.9393) -> (11.9697, -56.9697) projected
  line L69 (11.9697, -56.9697) -> (10, -55) projected
  line L70 (10, -55) -> (10, -33.5607) projected
  line L71 (10, -33.5607) -> (12.5, -31.0607) projected
  line L72 (12.5, -31.0607) -> (15, -33.5607) projected
  line L73 (15, -33.5607) -> (15, -53.9393) projected
  line L74 (13.0303, -58.0303) -> (16.0607, -55) projected
  line L75 (16.0607, -55) -> (33.9393, -55) projected
  line L76 (33.9393, -55) -> (36.9697, -58.0303) projected
  line L77 (36.9697, -58.0303) -> (35, -60) projected
  line L78 (35, -60) -> (15, -60) projected
  line L79 (15, -60) -> (13.0303, -58.0303) projected
  line L80 (38.0303, -56.9697) -> (35, -53.9393) projected
  line L81 (35, -53.9393) -> (35, -33.5607) projected
  line L82 (35, -33.5607) -> (37.5, -31.0607) projected
  line L83 (37.5, -31.0607) -> (40, -33.5607) projected
  line L84 (40, -33.5607) -> (40, -55) projected
  line L85 (40, -55) -> (38.0303, -56.9697) projected
  line L86 (16.0607, -27.5) -> (33.9393, -27.5) projected
  line L87 (33.9393, -27.5) -> (36.4393, -30) projected
  line L88 (36.4393, -30) -> (33.9393, -32.5) projected
  line L89 (33.9393, -32.5) -> (16.0607, -32.5) projected
  line L90 (16.0607, -32.5) -> (13.5607, -30) projected
  line L91 (13.5607, -30) -> (16.0607, -27.5) projected
  line L92 (11.9697, -3.0303) -> (15, -6.0607) projected
  line L93 (15, -6.0607) -> (15, -26.4393) projected
  line L94 (15, -26.4393) -> (12.5, -28.9393) projected
  line L95 (12.5, -28.9393) -> (10, -26.4393) projected
  line L96 (10, -26.4393) -> (10, -5) projected
  line L97 (10, -5) -> (11.9697, -3.0303) projected
  line L98 (16.0607, -5) -> (13.0303, -1.9697) projected
  line L99 (13.0303, -1.9697) -> (15, 0) projected
  line L100 (15, 0) -> (35, 0) projected
  line L101 (35, 0) -> (36.9697, -1.9697) projected
  line L102 (36.9697, -1.9697) -> (33.9393, -5) projected
  line L103 (33.9393, -5) -> (16.0607, -5) projected
  circle A0 centre (52.5, -15.7197) radius 4 projected
  circle A1 centre (52.5, -15.7197) radius 2.5 projected
  circle A2 centre (52.5, -44.2803) radius 2.5 projected
  circle A3 centre (52.5, -44.2803) radius 4 projected
  line L104 (148, 0) -> (148, -60) projected
  line L105 (131.5, -61.5) -> (131.5, 1.5) projected
  line L106 (63.5, 1.5) -> (63.5, -61.5) projected
  line L107 (150, -60) -> (150, 0) projected
  line L108 (-45, 0) -> (-45, -60) projected
  line L109 (-31.5, 3.5) -> (56.5, 3.5)
  line L110 (56.5, 3.5) -> (56.5, -63.5)
  line L111 (56.5, -63.5) -> (-31.5, -63.5)
  line L112 (-31.5, -63.5) -> (-31.5, 3.5)
  circle A4 centre (52.5, -0.5) radius 2.15
  circle A5 centre (52.5, -0.5) radius 4
  circle A6 centre (-27.5, -0.5) radius 4
  circle A7 centre (-27.5, -0.5) radius 2.15
  circle A8 centre (52.5, -59.5) radius 4
  circle A9 centre (52.5, -59.5) radius 2.15
  circle A10 centre (-27.5, -59.5) radius 4
  circle A11 centre (-27.5, -59.5) radius 2.15
  circle A12 centre (62.5, -0.5) radius 4
  circle A13 centre (62.5, -0.5) radius 2.15
  line L113 (58.5, 3.5) -> (146.5, 3.5)
  circle A14 centre (142.5, -0.5) radius 4
  circle A15 centre (142.5, -0.5) radius 2.15
  line L114 (146.5, 3.5) -> (146.5, -63.5)
  circle A16 centre (142.5, -59.5) radius 4
  circle A17 centre (142.5, -59.5) radius 2.15
  line L115 (146.5, -63.5) -> (58.5, -63.5)
  circle A18 centre (62.5, -59.5) radius 4
  circle A19 centre (62.5, -59.5) radius 2.15
  line L116 (58.5, -63.5) -> (58.5, 3.5)
  point P0 (115, -30)
  point P1 (-1.5, -16.25)
  point P2 (56.5, -30.7197)
  point P3 (-26.5, -30)
  point P4 (-31.5, -30)
  point P5 (58.5, -30)
  point P6 (63.5, 1.4033)
  point P7 (63.5, -2.4033)
  point P8 (63.5, -57.5967)
  point P9 (63.5, -61.4033)
  point P10 (-26.5, -57.5967)
  point P11 (-26.5, -61.4033)
  point P12 (-26.5, 1.4033)
  point P13 (-26.5, -2.4033)
  dimension "d104" = 68
  dimension "d105" = 63
  dimension "d107" = 17
  dimension "d108" = 19.5
  dimension "d109" = 15
  dimension "d110" = 16.5
  dimension "d112" = 195
  dimension "d114" = 7
  dimension "d115" = 5
  dimension "d116" = 67
  dimension "d117" = 88
  dimension "bobyshka_d" = 4.3
  dimension "d119" = 8
  dimension "d120" = 8
  dimension "d121" = 4.3
  dimension "d122" = 8
  dimension "d123" = 4.3
  dimension "d124" = 8
  dimension "d125" = 4.3
  dimension "d128" = 90
  constraints: 16 centre point, 16 end point, 9 tangent, 8 coincident, 3 midpoint, 2 horizontal, 2 parallel, 1 collinear, 1 horizontal alignment, 1 perpendicular, 24 other
  measures "d104" distance between parallel lines of L17 L19
  measures "d105" distance of L18.end L16.start
  measures "d107" distance from line of point (-1.5, -16.25) L10
  measures "d108" distance between parallel lines of L9 L11
  measures "d109" distance from line of point (56.5, -30.72) L17
  measures "d110" distance between parallel lines of L104 L105
  measures "d112" distance between parallel lines of L107 L108
  measures "d114" distance between parallel lines of L106 L110
  measures "d115" distance between parallel lines of L112 L19
  measures "d116" distance of L111.end L109.start
  measures "d117" distance of L109.start L109.end
  measures "bobyshka_d" diameter of A4
  measures "d119" diameter of A5
  measures "d120" diameter of A6
  measures "d121" diameter of A7
  measures "d122" diameter of A8
  measures "d123" diameter of A9
  measures "d124" diameter of A10
  measures "d125" diameter of A11
  measures "d128" distance of A6.centre A12.centre
extrude "Extrusion5" add sketch "Sketch5" against normal up to surface (7 mm away) contours L19 A11 A10 L16 | L16 A10 L19 A11 | A8 | A6 L19 A7 L18 | L18 L19 A7 A6 | A5 | A12 | A18 | A14 | A16
extrude "Extrusion6" cut sketch "Sketch5" against normal up to surface (7 mm away) contours L19 A11 | L19 A7 | A13 L106 | A19 L106 picked at (-26.1167, -59.5) picked at (-26.1167, -0.5) picked at (64.1027, -0.4551) picked at (64.1027, -59.4551)
sketch "Sketch8" plane through (115, 30, -7.5) normal (0, 0, -1) x (-1, 0, 0)
  circle A0 centre (-27.5, -0.5) radius 2.15 projected
  circle A1 centre (-27.5, -59.5) radius 2.15 projected
  arc A2 (-24.0359, 1.5) -> (-26.5, -4.373) centre (-27.5, -0.5) ccw projected
  line L0 (-26.5, -4.373) -> (-26.5, -55.627) projected
  arc A3 (-26.5, -55.627) -> (-24.0359, -61.5) centre (-27.5, -59.5) ccw projected
  line L1 (-24.0359, -61.5) -> (41.5, -61.5) projected
  line L2 (41.5, -61.5) -> (41.5, 1.5) projected
  line L3 (41.5, 1.5) -> (-24.0359, 1.5) projected
  line L4 (16.0607, -5) -> (13.0303, -1.9697) projected
  line L5 (13.0303, -1.9697) -> (15, 0) projected
  line L6 (15, 0) -> (35, 0) projected
  line L7 (35, 0) -> (36.9697, -1.9697) projected
  line L8 (36.9697, -1.9697) -> (33.9393, -5) projected
  line L9 (33.9393, -5) -> (16.0607, -5) projected
  line L10 (11.9697, -3.0303) -> (15, -6.0607) projected
  line L11 (15, -6.0607) -> (15, -26.4393) projected
  line L12 (15, -26.4393) -> (12.5, -28.9393) projected
  line L13 (12.5, -28.9393) -> (10, -26.4393) projected
  line L14 (10, -26.4393) -> (10, -5) projected
  line L15 (10, -5) -> (11.9697, -3.0303) projected
  line L16 (16.0607, -27.5) -> (33.9393, -27.5) projected
  line L17 (33.9393, -27.5) -> (36.4393, -30) projected
  line L18 (36.4393, -30) -> (33.9393, -32.5) projected
  line L19 (33.9393, -32.5) -> (16.0607, -32.5) projected
  line L20 (16.0607, -32.5) -> (13.5607, -30) projected
  line L21 (13.5607, -30) -> (16.0607, -27.5) projected
  line L22 (38.0303, -56.9697) -> (35, -53.9393) projected
  line L23 (35, -53.9393) -> (35, -33.5607) projected
  line L24 (35, -33.5607) -> (37.5, -31.0607) projected
  line L25 (37.5, -31.0607) -> (40, -33.5607) projected
  line L26 (40, -33.5607) -> (40, -55) projected
  line L27 (40, -55) -> (38.0303, -56.9697) projected
  line L28 (13.0303, -58.0303) -> (16.0607, -55) projected
  line L29 (16.0607, -55) -> (33.9393, -55) projected
  line L30 (33.9393, -55) -> (36.9697, -58.0303) projected
  line L31 (36.9697, -58.0303) -> (35, -60) projected
  line L32 (35, -60) -> (15, -60) projected
  line L33 (15, -60) -> (13.0303, -58.0303) projected
  line L34 (15, -53.9393) -> (11.9697, -56.9697) projected
  line L35 (11.9697, -56.9697) -> (10, -55) projected
  line L36 (10, -55) -> (10, -33.5607) projected
  line L37 (10, -33.5607) -> (12.5, -31.0607) projected
  line L38 (12.5, -31.0607) -> (15, -33.5607) projected
  line L39 (15, -33.5607) -> (15, -53.9393) projected
  line L40 (3.0303, -56.9697) -> (0, -53.9393) projected
  line L41 (0, -53.9393) -> (0, -33.5607) projected
  line L42 (0, -33.5607) -> (2.5, -31.0607) projected
  line L43 (2.5, -31.0607) -> (5, -33.5607) projected
  line L44 (5, -33.5607) -> (5, -55) projected
  line L45 (5, -55) -> (3.0303, -56.9697) projected
  line L46 (-18.9393, -27.5) -> (-1.0607, -27.5) projected
  line L47 (-1.0607, -27.5) -> (1.4393, -30) projected
  line L48 (1.4393, -30) -> (-1.0607, -32.5) projected
  line L49 (-1.0607, -32.5) -> (-18.9393, -32.5) projected
  line L50 (-18.9393, -32.5) -> (-21.4393, -30) projected
  line L51 (-21.4393, -30) -> (-18.9393, -27.5) projected
  line L52 (0, -6.0607) -> (3.0303, -3.0303) projected
  line L53 (3.0303, -3.0303) -> (5, -5) projected
  line L54 (5, -5) -> (5, -26.4393) projected
  line L55 (5, -26.4393) -> (2.5, -28.9393) projected
  line L56 (2.5, -28.9393) -> (0, -26.4393) projected
  line L57 (0, -26.4393) -> (0, -6.0607) projected
  line L58 (-18.9393, -5) -> (-21.9697, -1.9697) projected
  line L59 (-21.9697, -1.9697) -> (-20, 0) projected
  line L60 (-20, 0) -> (0, 0) projected
  line L61 (0, 0) -> (1.9697, -1.9697) projected
  line L62 (1.9697, -1.9697) -> (-1.0607, -5) projected
  line L63 (-1.0607, -5) -> (-18.9393, -5) projected
  line L64 (-20, -53.9393) -> (-23.0303, -56.9697) projected
  line L65 (-23.0303, -56.9697) -> (-25, -55) projected
  line L66 (-25, -55) -> (-25, -33.5607) projected
  line L67 (-25, -33.5607) -> (-22.5, -31.0607) projected
  line L68 (-22.5, -31.0607) -> (-20, -33.5607) projected
  line L69 (-20, -33.5607) -> (-20, -53.9393) projected
  line L70 (-21.9697, -58.0303) -> (-18.9393, -55) projected
  line L71 (-18.9393, -55) -> (-1.0607, -55) projected
  line L72 (-1.0607, -55) -> (1.9697, -58.0303) projected
  line L73 (1.9697, -58.0303) -> (0, -60) projected
  line L74 (0, -60) -> (-20, -60) projected
  line L75 (-20, -60) -> (-21.9697, -58.0303) projected
  line L76 (38.0303, -3.0303) -> (40, -5) projected
  line L77 (40, -5) -> (40, -26.4393) projected
  line L78 (40, -26.4393) -> (37.5, -28.9393) projected
  line L79 (37.5, -28.9393) -> (35, -26.4393) projected
  line L80 (35, -26.4393) -> (35, -6.0607) projected
  line L81 (35, -6.0607) -> (38.0303, -3.0303) projected
  line L82 (-22.5, -28.9393) -> (-25, -26.4393) projected
  line L83 (-25, -26.4393) -> (-25, -5) projected
  line L84 (-25, -5) -> (-23.0303, -3.0303) projected
  line L85 (-23.0303, -3.0303) -> (-20, -6.0607) projected
  line L86 (-20, -6.0607) -> (-20, -26.4393) projected
  line L87 (-20, -26.4393) -> (-22.5, -28.9393) projected
  line L88 (33.5, -6.5) -> (33.5, -26) projected
  line L89 (33.5, -26) -> (16.5, -26) projected
  line L90 (16.5, -26) -> (16.5, -6.5) projected
  line L91 (16.5, -6.5) -> (33.5, -6.5) projected
  line L92 (-1.5, -6.5) -> (-1.5, -26) projected
  line L93 (-1.5, -26) -> (-18.5, -26) projected
  line L94 (-18.5, -26) -> (-18.5, -6.5) projected
  line L95 (-18.5, -6.5) -> (-1.5, -6.5) projected
  line L96 (33.5, -53.5) -> (16.5, -53.5) projected
  line L97 (16.5, -53.5) -> (16.5, -34) projected
  line L98 (16.5, -34) -> (33.5, -34) projected
  line L99 (33.5, -34) -> (33.5, -53.5) projected
  line L100 (-1.5, -53.5) -> (-18.5, -53.5) projected
  line L101 (-18.5, -53.5) -> (-18.5, -34) projected
  line L102 (-18.5, -34) -> (-1.5, -34) projected
  line L103 (-1.5, -34) -> (-1.5, -53.5) projected
  circle A4 centre (52.5, -0.5) radius 4 projected
  circle A5 centre (52.5, -0.5) radius 2.15 projected
  circle A6 centre (52.5, -15.7197) radius 4 projected
  circle A7 centre (52.5, -15.7197) radius 2.5 projected
  circle A8 centre (52.5, -44.2803) radius 2.5 projected
  circle A9 centre (52.5, -44.2803) radius 4 projected
  circle A10 centre (52.5, -59.5) radius 4 projected
  circle A11 centre (52.5, -59.5) radius 2.15 projected
  line L104 (-31.5, 3.5) -> (56.5, 3.5)
  line L105 (56.5, 3.5) -> (56.5, -63.5)
  line L106 (56.5, -63.5) -> (-31.5, -63.5)
  line L107 (-31.5, -63.5) -> (-31.5, 3.5)
  circle A12 centre (52.5, -59.5) radius 4 projected
  arc A13 (-24.0359, 1.5) -> (-26.5, -4.373) centre (-27.5, -0.5) ccw projected
  line L108 (-15.5, -5) -> (-4.5, -5)
  line L109 (-4.5, -5) -> (-4.5, 0)
  line L110 (-4.5, 0) -> (-15.5, 0)
  line L111 (-15.5, 0) -> (-15.5, -5)
  circle A14 centre (-15.5, -2.5) radius 2
  circle A15 centre (-4.5, -2.5) radius 2
  line L112 (30.5, -5) -> (30.5, 0)
  line L113 (19.5, -5) -> (30.5, -5)
  line L114 (30.5, 0) -> (19.5, 0)
  line L115 (19.5, 0) -> (19.5, -5)
  circle A16 centre (19.5, -2.5) radius 2
  circle A17 centre (30.5, -2.5) radius 2
  line L116 (-4.5, -32.5) -> (-4.5, -27.5)
  line L117 (-15.5, -32.5) -> (-4.5, -32.5)
  line L118 (-4.5, -27.5) -> (-15.5, -27.5)
  line L119 (-15.5, -27.5) -> (-15.5, -32.5)
  circle A18 centre (-15.5, -30) radius 2
  circle A19 centre (-4.5, -30) radius 2
  line L120 (30.5, -32.5) -> (30.5, -27.5)
  line L121 (19.5, -32.5) -> (30.5, -32.5)
  line L122 (30.5, -27.5) -> (19.5, -27.5)
  line L123 (19.5, -27.5) -> (19.5, -32.5)
  circle A20 centre (19.5, -30) radius 2
  circle A21 centre (30.5, -30) radius 2
  line L124 (-4.5, -60) -> (-4.5, -55)
  line L125 (-15.5, -60) -> (-4.5, -60)
  line L126 (-4.5, -55) -> (-15.5, -55)
  line L127 (-15.5, -55) -> (-15.5, -60)
  circle A22 centre (-15.5, -57.5) radius 2
  circle A23 centre (-4.5, -57.5) radius 2
  line L128 (30.5, -60) -> (30.5, -55)
  line L129 (19.5, -60) -> (30.5, -60)
  line L130 (30.5, -55) -> (19.5, -55)
  line L131 (19.5, -55) -> (19.5, -60)
  circle A24 centre (19.5, -57.5) radius 2
  circle A25 centre (30.5, -57.5) radius 2
  line L132 (-20, -26.4393) -> (-20, -6.0607) projected
  line L133 (-25, -9.2197) -> (-20, -9.2197)
  line L134 (-20, -9.2197) -> (-20, -22.2197)
  line L135 (-20, -22.2197) -> (-25, -22.2197)
  line L136 (-25, -22.2197) -> (-25, -9.2197)
  circle A26 centre (-22.5, -9.2197) radius 2
  circle A27 centre (-22.5, -22.2197) radius 2
  circle A28 centre (-22.5, -37.7807) radius 2
  circle A29 centre (-22.5, -50.7807) radius 2
  circle A30 centre (2.522, -9.2197) radius 2
  circle A31 centre (2.522, -22.2197) radius 2
  circle A32 centre (2.522, -37.7807) radius 2
  circle A33 centre (2.522, -50.7807) radius 2
  circle A34 centre (37.522, -22.2197) radius 2
  circle A35 centre (12.5, -9.2197) radius 2
  circle A36 centre (37.522, -9.2197) radius 2
  circle A37 centre (12.5, -22.2197) radius 2
  circle A38 centre (12.5, -37.7807) radius 2
  circle A39 centre (12.5, -50.7807) radius 2
  circle A40 centre (37.522, -37.7807) radius 2
  circle A41 centre (37.522, -50.7807) radius 2
  line L137 (-22.5, -9.2197) -> (-22.5, -22.2197)
  line L138 (-15.5, -2.5) -> (-4.5, -2.5)
  line L139 (-22.5, -37.7807) -> (-22.5, -50.7807)
  line L140 (-15.5, -30) -> (-4.5, -30)
  line L141 (2.522, -9.2197) -> (2.522, -22.2197)
  line L142 (2.522, -37.7807) -> (2.522, -50.7807)
  line L143 (-15.5, -57.5) -> (-4.5, -57.5)
  circle A42 centre (-22.5, -15.7197) radius 1.5
  circle A43 centre (-10, -2.5) radius 1.5
  circle A44 centre (2.522, -15.7197) radius 1.5
  circle A45 centre (-22.5, -44.2807) radius 1.5
  circle A46 centre (2.522, -44.2807) radius 1.5
  circle A47 centre (-10, -30) radius 1.5
  circle A48 centre (-10, -57.5) radius 1.5
  circle A49 centre (12.5, -15.7197) radius 1.5
  circle A50 centre (25, -2.5) radius 1.5
  circle A51 centre (37.522, -15.7197) radius 1.5
  circle A52 centre (25, -30) radius 1.5
  circle A53 centre (12.5, -44.2807) radius 1.5
  circle A54 centre (25, -57.5) radius 1.5
  circle A55 centre (37.522, -44.2807) radius 1.5
  point P0 (115, -30)
  point P1 (-10, 0)
  point P2 (25, 0)
  point P3 (-10, -27.5)
  point P4 (25, -27.5)
  point P5 (-10, -55)
  point P6 (25, -55)
  point P7 (-25, -15.7197)
  dimension "d141" = 22.8787
  dimension "d142" = 25.909
  dimension "d143" = 11
  dimension "d144" = 4
  dimension "d145" = 4
  dimension "d148" = 35
  dimension "d151" = 27.5
  dimension "d161" = 13
  dimension "d162" = 4
  dimension "d163" = 4
  dimension "d166" = 28.561
  dimension "d169" = 25.022
  dimension "d174" = 35
  dimension "d186" = 3
  dimension "d187" = 3
  dimension "d188" = 3
  dimension "d189" = 3
  dimension "d190" = 3
  dimension "d191" = 3
  dimension "d192" = 3
  dimension "d195" = 35
  dimension "d200" = 88
  dimension "d201" = 67
  constraints: 78 end point, 42 centre point, 15 midpoint, 8 coincident, 8 horizontal, 8 parallel, 5 vertical, 4 perpendicular, 4 point on line, 4 tangent, 112 other
  measures "d141" distance of L50.end L47.end
  measures "d142" vertical distance of L84.end L82.start
  measures "d143" distance from line of L109 point (-15.5, -2.5)
  measures "d144" diameter of A14
  measures "d145" diameter of A15
  measures "d148" distance of L109.end L112.end
  measures "d151" distance of L109.end L116.end
  measures "d161" distance of point (-22.5, -9.22) point (-22.5, -22.22)
  measures "d162" diameter of A26
  measures "d163" diameter of A27
  measures "d166" distance of L137.start L139.start
  measures "d169" distance of L137.start L141.start
  measures "d174" distance of L141.end A34.centre
  measures "d186" diameter of A42
  measures "d187" diameter of A43
  measures "d188" diameter of A44
  measures "d189" diameter of A45
  measures "d190" diameter of A46
  measures "d191" diameter of A47
  measures "d192" diameter of A48
  measures "d195" distance of A42.centre A49.centre
  measures "d200" distance of L104.start L104.end
  measures "d201" distance of L104.end L105.end
fillet "Fillet1" radius 4 4 edges at (73.5, 31.5, -4) (-16.5, 31.5, -4) (-16.5, -31.5, -4) (73.5, -31.5, -4)
equation "\"d121\" = bobyshka_d"
equation "\"d123\" = bobyshka_d"
equation "\"d125\" = bobyshka_d"
body "Solid1"
